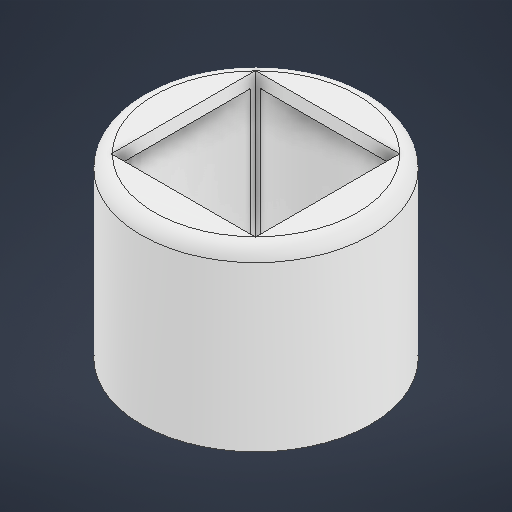
# Autodesk Inventor part: module
Saved by Autodesk Inventor 2026.2 (Build 302298000, 298)
## iProperties
Created: 2026-04-08
Part Number: module
Material: ABS Plastic
Document SubType Name: Modeling
Designer: Koda
Density: 1.06 g/cm^3
Appearance: Smooth - White
Author: Koda
Autodesk Inventor part; units mm, degrees
ref_plane "YZ Plane" through (0, 0, 0) normal (1, 0, 0) x (0, 1, 0)
ref_plane "XZ Plane" through (0, 0, 0) normal (0, 1, 0) x (-1, 0, 0)
ref_plane "XY Plane" through (0, 0, 0) normal (0, 0, 1) x (1, 0, 0)
sketch "Sketch1" plane through (0, 0, 0) normal (0, 1, 0) x (-1, 0, 0)
  circle A0 centre (0, 0) radius 22.225
  dimension "d0" = 44.45
  constraints: 1 centre point, 1 coincident
  measures "d0" diameter of A0
extrude "Extrusion1" add sketch "Sketch1" along normal blind 34.29
fillet "Fillet1" radius 2.54 1 edges at (22.225, 34.29, 0)
sketch "Sketch2" plane through (0, 0, 0) normal (0, -1, 0) x (1, 0, 0)
  circle A0 centre (0, 0) radius 19.05
  dimension "d4" = 38.1
  constraints: 1 centre point, 1 coincident
  measures "d4" diameter of A0
extrude "Extrusion2" cut sketch "Sketch2" against normal blind 31.75
sketch "Sketch3" plane through (0, 34.29, 0) normal (0, 1, 0) x (1, 0, 0)
  line L0 (0, 0) -> (0, -13.97)
  line L1 (0, 0) -> (-13.97, 0)
  line L2 (-14.0204, -14.0204) -> (13.9196, -14.0204)
  line L3 (13.9196, -14.0204) -> (13.9196, 13.9196)
  line L4 (13.9196, 13.9196) -> (-14.0204, 13.9196)
  line L5 (-14.0204, 13.9196) -> (-14.0204, -14.0204)
  dimension "d7" = 13.97
  dimension "d8" = 13.97
  dimension "d9" = 27.94
  dimension "d10" = 27.94
  constraints: 12 end point, 2 horizontal, 2 parallel, 1 perpendicular, 1 vertical
  measures "d7" distance of L0.start L0.end
  measures "d8" distance of L0.start L1.end
  measures "d9" distance of L4.end L3.end
  measures "d10" distance of L3.end L2.end
extrude "Extrusion3" cut sketch "Sketch3" against normal blind 31.75
sketch "Sketch4" plane through (0, 0, 0) normal (0, -1, 0) x (1, 0, 0)
  line L0 (13.8176, 14.0204) -> (-13.8176, 14.0204) projected
  line L1 (0, 14.0204) -> (-12.8969, 14.0204)
  arc A0 (13.9196, -13.0057) -> (13.9196, 13.0057) centre (0, 0) ccw projected
  line L2 (0, 14.0204) -> (12.8969, 14.0204)
  circle A1 centre (0, 0) radius 19.05
  point P0 (10.16, 10.16)
  point P1 (-10.16, 10.16)
  point P2 (12.8969, 14.0204)
  point P3 (-12.8969, 14.0204)
  point P4 (-13.8176, 14.0204)
  constraints: 4 end point, 2 point on circle, 1 centre point, 1 coincident, 1 concentric, 1 horizontal, 1 point on line, 2 other
extrude "Extrusion4" add sketch "Sketch4" against normal blind 34.29 contours L0 A1
body "Solid1"
